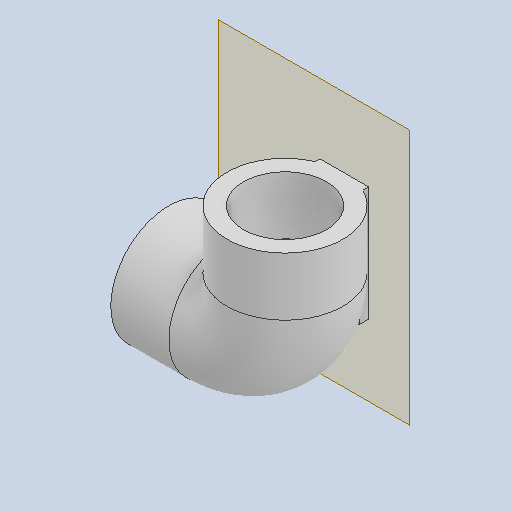
# Autodesk Inventor part: Knee
Saved by Autodesk Inventor 2025 (Build 290162000, 162)
## iProperties
Created: 2025-07-16
Part Number: Knee
Material: Generic
Document SubType Name: Modeling
Designer: Pravoslav
Density: 1 g/cm^3
Appearance: Default
Author: Pravoslav
Autodesk Inventor part; units mm, degrees
ref_plane "YZ Plane" through (0, 0, 0) normal (1, 0, 0) x (0, 1, 0)
sketch "Sketch1" plane through (0, 0, 0) normal (0, 1, 0) x (-1, 0, 0)
  circle A0 centre (0, 0) radius 5
  circle A1 centre (0, 0) radius 3.575
  line L0 (5, 0) -> (5, -7.589)
  dimension "d0" = 10
  dimension "d1" = 7.15
  constraints: 2 coincident, 2 end point, 2 vertical, 1 centre point, 1 horizontal alignment, 2 other
  measures "d1" diameter of A1
revolve "Revolution1" add sketch "Sketch1" angle 90 about axis through (-5, 0, 0) along (0, 0, -1)
sketch "Sketch3" plane through (-5, -5, 0) normal (-1, 0, 0) x (0, 0, 1)
  circle A0 centre (0, 0) radius 3.575
  circle A1 centre (0, 0) radius 5
  point P0 (0, 5)
  dimension "d8" = 7.15
  dimension "d9" = 10
  constraints: 2 centre point, 1 coincident
  measures "d8" diameter of A0
  measures "d9" diameter of A1
extrude "Extrusion1" add sketch "Sketch3" along normal blind 5
sketch "Sketch4" plane through (0, 0, 0) normal (0, 1, 0) x (1, 0, 0)
  circle A0 centre (0, 0) radius 3.575
  circle A1 centre (0, 0) radius 5
  dimension "d12" = 7.15
  dimension "d13" = 10
  constraints: 2 centre point, 2 coincident
  measures "d12" diameter of A0
  measures "d13" diameter of A1
extrude "Extrusion2" add sketch "Sketch4" along normal blind 5
ref_plane "Work Plane3" through (-5, -5, -5) normal (0, 0, 1) x (1, 0, 0)
sketch "Sketch5" plane through (-5, -5, -5) normal (0, 0, 1) x (1, 0, 0)
  line L0 (1.425, 10) -> (8.575, 10) projected
  line L1 (7.1875, 10) -> (3.0146, 10)
  line L2 (3.0146, 10) -> (3.0146, 0.1288)
  line L3 (3.0146, 0.1288) -> (7.1875, 0.1288)
  line L4 (7.1875, 0.1288) -> (7.1875, 10)
  line L5 (-5, -3.575) -> (-5, 3.575) projected
  line L6 (-5, 1.9486) -> (4.7301, 1.9486)
  line L7 (4.7301, 1.9486) -> (4.7301, -1.691)
  line L8 (4.7301, -1.691) -> (-5, -1.691)
  line L9 (-5, -1.691) -> (-5, 1.9486)
  line L10 (4.7301, -1.691) -> (7.1875, 0.1288)
  point P0 (5, 5)
  point P1 (3.0146, 1.9486)
  dimension "d4" = 10
  dimension "d5" = 5
  dimension "d6" = 7.15
  constraints: 18 end point, 4 parallel, 2 horizontal, 2 perpendicular, 2 point on line
extrude "Extrusion3" add sketch "Sketch5" along normal blind 0.75
ref_plane "Work Plane1" through (0, 0, 0) normal (0, 0, 1) x (1, 0, 0)
body "Solid1"
